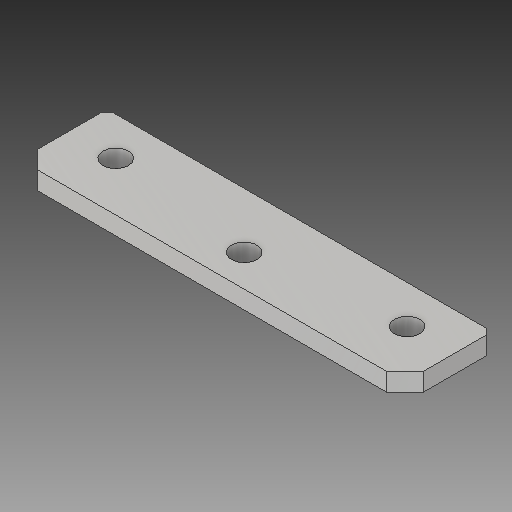
# Autodesk Inventor part: stopperver2_1
Saved by Autodesk Inventor 2018 (Build 220112000, 112)
## iProperties
Created: 2020-08-12
Part Number: stopperver2_1
Material: 一般
Document SubType Name: Modeling
Designer: gisen
Density: 1 g/cm^3
Appearance: 機械加工 - アルミニウム
Mass: 2.62931 g
Surface Area: 23.2857 cm^2
Volume: 2.62931 cm^3
Author: gisen
Autodesk Inventor part; units mm, degrees
ref_plane "YZ Plane" through (0, 0, 0) normal (1, 0, 0) x (0, 1, 0)
ref_plane "XZ Plane" through (0, 0, 0) normal (0, 1, 0) x (-1, 0, 0)
ref_plane "XY Plane" through (0, 0, 0) normal (0, 0, 1) x (1, 0, 0)
sketch "スケッチ1" plane through (0, 0, 0) normal (0, 1, 0) x (-1, 0, 0)
  circle A0 centre (55.3, 11.85) radius 2.1
  circle A1 centre (31.1, 14.7) radius 2.1
  circle A2 centre (6.9, 11.85) radius 2.1
  line L0 (62.1, 5.5) -> (0.1, 5.5)
  line L1 (2.1, 20) -> (60.1, 20)
  line L2 (2.1, 20) -> (18.1, 20)
  line L3 (-0.9, 6.5) -> (-0.9, 17)
  line L4 (63.1, 17) -> (63.1, 6.5)
  line L5 (63.1, 17) -> (60.1, 20)
  line L6 (-0.9, 17) -> (2.1, 20)
  line L7 (63.1, 6.5) -> (62.1, 5.5)
  line L8 (0.1, 5.5) -> (-0.9, 6.5)
  point P0 (0, 0)
  point P1 (-0.9, 5.5)
  point P2 (-0.9, 20)
  point P3 (63.1, 20)
  point P4 (63.1, 5.5)
  dimension "d0" = 64
  dimension "d2" = 14.5
  dimension "d3" = 4.2
  dimension "d4" = 4.2
  dimension "d5" = 4.2
  dimension "d8" = 3
  dimension "d9" = 3
  dimension "d10" = 3
  dimension "d11" = 3
  dimension "d12" = 1
  dimension "d13" = 1
  dimension "d14" = 1
  dimension "d15" = 1
  constraints: 18 end point, 8 point on line, 3 centre point
  measures "d0" distance between parallel lines of L3 L4
  measures "d2" distance between parallel lines of L1 L0
  measures "d3" diameter of A0
  measures "d4" diameter of A1
  measures "d5" diameter of A2
  measures "d8" distance of L4.start point (63.1, 20)
  measures "d9" distance of L1.end point (63.1, 20)
  measures "d10" distance of L3.end point (-0.9, 20)
  measures "d11" distance of L1.start point (-0.9, 20)
  measures "d12" distance of L4.end point (63.1, 5.5)
  measures "d13" distance of L0.start point (63.1, 5.5)
  measures "d14" distance of L0.end point (-0.9, 5.5)
  measures "d15" distance of L3.start point (-0.9, 5.5)
extrude "押し出し1" add sketch "スケッチ1" along normal blind 3
equation "\"d4\" = d3"
equation "\"d5\" = d4"
equation "\"d9\" = d8"
equation "\"d10\" = d8"
equation "\"d11\" = d10"
equation "\"d13\" = d12"
equation "\"d14\" = d12"
equation "\"d15\" = d14"
